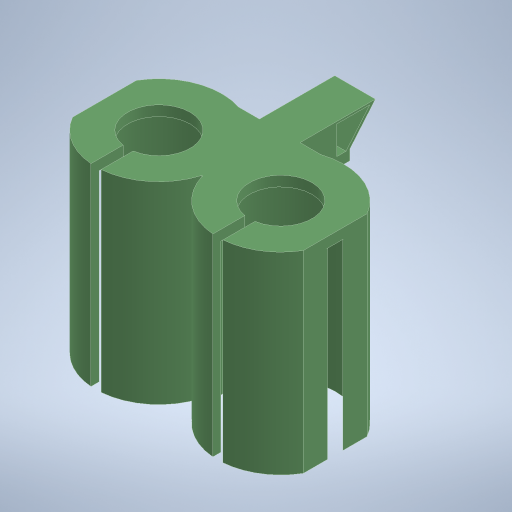
# Autodesk Inventor part: vialHolder_2v
Saved by Autodesk Inventor 2023.4 (Build 274418000, 418)
## iProperties
Created: 2023-09-01
Part Number: vialHolder_2v
Material: Generic
Document SubType Name: Modeling
Designer: SB13FLLT004
Density: 1 g/cm^3
Appearance: Dark Green(3)
Author: SB13FLLT004
Autodesk Inventor part; units mm, degrees
ref_plane "YZ Plane" through (0, 0, 0) normal (1, 0, 0) x (0, 1, 0)
ref_plane "XZ Plane" through (0, 0, 0) normal (0, 1, 0) x (-1, 0, 0)
ref_plane "XY Plane" through (0, 0, 0) normal (0, 0, 1) x (1, 0, 0)
derived "main_manifold_8v_v02.ipt"
sketch "Sketch:MM: flow sensor" plane through (0, 0, -27.94) normal (0, -1, 0) x (1, 0, 0)
  line L0 (19.2278, 23.241) -> (22.6822, 23.241)
  line L1 (49.7078, 23.241) -> (53.1622, 23.241)
  line L2 (110.6678, 23.241) -> (114.1222, 23.241)
  line L3 (80.1878, 23.241) -> (83.6422, 23.241)
  line L4 (141.1478, 23.241) -> (144.6022, 23.241)
  line L5 (171.6278, 23.241) -> (175.0822, 23.241)
  line L6 (202.1078, 23.241) -> (205.5622, 23.241)
  line L7 (232.5878, 23.241) -> (236.0422, 23.241)
  line L8 (0, 27.94) -> (247.65, 27.94)
  point P0 (20.955, 23.241)
  point P1 (51.435, 23.241)
  point P2 (51.435, 23.241)
  point P3 (20.955, 23.241)
  point P4 (81.915, 23.241)
  point P5 (112.395, 23.241)
  point P6 (81.915, 23.241)
  point P7 (112.395, 23.241)
  point P8 (142.875, 23.241)
  point P9 (173.355, 23.241)
  point P10 (203.835, 23.241)
  point P11 (234.315, 23.241)
  point P12 (142.875, 23.241)
  point P13 (173.355, 23.241)
  point P14 (203.835, 23.241)
  point P15 (234.315, 23.241)
derived "vial_ST_01.ipt"
derived "mainPlate.ipt"
sketch "Sketch:VH: vials" plane through (0, 0, 0) normal (0, 1, 0) x (-1, 0, 0)
  circle A0 centre (-20.955, -4.699) radius 15.7798
  circle A1 centre (-20.955, -4.699) radius 13.7477
  circle A2 centre (-20.955, -4.699) radius 7.5565 construction
  circle A3 centre (-20.955, -4.699) radius 7.8105
  circle A4 centre (-51.435, -4.699) radius 15.7798
  circle A5 centre (-51.435, -4.699) radius 13.7477
  circle A6 centre (-51.435, -4.699) radius 7.8105
  line L0 (-36.0958, -9.144) -> (-36.2942, -9.144)
  line L1 (-36.0958, -0.254) -> (-36.2942, -0.254)
  point P0 (0, 0)
  point P1 (-36.195, -0.6072)
  point P2 (-36.195, -8.7908)
  dimension "cap_diameter" = 15.113
  dimension "d5" = 15.621
  dimension "extra_space_around_vial_front_and_back" = 4.445
  constraints: 7 centre point, 7 coincident, 4 end point, 4 point on circle, 3 equal radius, 2 vertical alignment, 1 concentric, 1 horizontal, 1 horizontal alignment, 1 other
  measures "cap_diameter" diameter of A2
  measures "d5" diameter of A3
  measures "extra_space_around_vial_front_and_back" vertical distance of A0.centre L1.start
sketch "Sketch:VH: side cutout" plane through (0, 0, 0) normal (0, 1, 0) x (-1, 0, 0)
  line L0 (-7.3399, -12.6758) -> (-7.3399, 3.2778)
  line L1 (-65.0501, -12.6758) -> (-65.0501, 3.2778)
  circle A0 centre (-51.435, -4.699) radius 15.7798 projected
  circle A1 centre (-51.435, -4.699) radius 13.7477 projected
  circle A2 centre (-20.955, -4.699) radius 15.7798 projected
  circle A3 centre (-20.955, -4.699) radius 13.7477 projected
  line L2 (-5.4104, -7.4129) -> (-7.4778, -7.4129) construction
  line L3 (-5.4104, -1.9851) -> (-7.4778, -1.9851) construction
  line L4 (-7.4778, -7.4129) -> (-7.4778, -1.9851) construction
  point P0 (0, 0)
  point P1 (-7.3399, -6.604)
  point P2 (-7.3399, -2.794)
  point P3 (-7.4778, -4.699)
  dimension "d12" = 13.6151
  dimension "d57" = 3.81
  dimension "d58" = 5.4278
  constraints: 10 end point, 10 point on circle, 3 horizontal alignment, 2 point on line, 1 midpoint, 1 parallel, 1 perpendicular, 1 vertical
  measures "d12" distance from line of A2.centre L0
  measures "d57" distance of A3.end A3.start
  measures "d58" distance of L2.end L3.end
extrude "Ex: top of vials" add sketch "Sketch:VH: vials" along normal blind 2.54 contours A0 A4 | A0 A4 L1 | L0 A4 A0 | A4 A0 | A0 A4 | A1 | A5
extrude "Ex: around vials" add sketch "Sketch:VH: vials" against normal blind 45.72 contours A0 A4 | A0 A4 L1 | L0 A4 A0 | A4 A0 | A0 A4
extrude "Ex: side cutout" cut sketch "Sketch:VH: side cutout" along normal through all both and the other way through all contours L0 A3 A2 | L0 A3 | A0 L1 A1 | A1 L1 picked at (-7.3154, -5.1231) picked at (-65.0894, -4.4867)
sketch "Sketch:VH: screw part" plane through (0, 2.54, 0) normal (0, 1, 0) x (-1, 0, 0)
  circle A0 centre (-20.955, -4.699) radius 15.7798 projected
  circle A1 centre (-51.435, -4.699) radius 15.7798 projected
  line L0 (-16.0074, -19.6831) -> (-56.3826, -19.6831)
  line L1 (-36.0958, -9.144) -> (-36.2942, -9.144) projected
  line L2 (-31.115, -19.6831) -> (-31.115, -28.916)
  line L3 (-31.115, -28.916) -> (-41.275, -28.916)
  line L4 (-41.275, -28.916) -> (-41.275, -19.6831)
  line L5 (-33.9979, -28.916) -> (-38.3921, -28.916) construction
  line L6 (-38.3921, -28.916) -> (-38.3921, -23.582) construction
  line L7 (-38.3921, -23.582) -> (-33.9979, -23.582) construction
  line L8 (-33.9979, -23.582) -> (-33.9979, -28.916) construction
  point P0 (0, 0)
  point P1 (-36.195, -19.6831)
  point P2 (-36.195, -9.144)
  point P3 (-36.195, -28.916)
  point P4 (-25.9026, -19.6831)
  point P5 (-46.4874, -19.6831)
  dimension "d15" = 10.16
  dimension "d18" = 9.2329
  constraints: 16 end point, 6 perpendicular, 4 midpoint, 3 vertical alignment, 2 horizontal, 2 point on circle, 2 point on line, 1 collinear, 1 horizontal alignment
  measures "d15" distance of L2.end L3.end
  measures "d18" distance of L3.end L4.end
extrude "Ex: screw area" add sketch "Sketch:VH: screw part" against normal blind 7.62 contours L0 A1 L1 A0 | L2 L3 L4 L0
sketch "Sketch:VH: screw hole" plane through (41.275, 2.54, -28.916) normal (0, 0, -1) x (-1, 0, 0)
  line L0 (0, 0) -> (10.16, 0) projected
  line L1 (10.16, -7.62) -> (0, -7.62) projected
  line L2 (0, -7.62) -> (0, -7.62)
  line L3 (0, -7.62) -> (10.16, -7.62)
  line L4 (10.16, -7.62) -> (10.16, -7.62)
  point P0 (41.275, -2.54)
  point P1 (5.08, -3.175)
  point P2 (5.08, 0)
  dimension "d72" = 3.175
  dimension "screwhole_to_btm_of_MP" = 4.445
  constraints: 6 end point, 2 perpendicular, 1 collinear, 1 midpoint, 1 vertical alignment
  measures "d72" distance from line of L0 point (5.08, -3.175)
  measures "screwhole_to_btm_of_MP" distance from line of L3 point (5.08, -3.175)
hole "Hole: screw to MP" at (36.195, -0.635, -28.916) direction (0, 0, 1) diameter 4.3942 depth 5.334
sketch "Sketch:VH: extend front" plane through (0, 0, 0) normal (0, 1, 0) x (-1, 0, 0)
  arc A0 (-7.3399, 4.2408) -> (-36.6245, -0.254) centre (-20.955, -4.699) ccw
  circle A1 centre (-20.955, -4.699) radius 15.7798 projected
  line L0 (-7.3399, -12.6758) -> (-7.3399, 3.2778) projected
  line L1 (-36.0958, -0.254) -> (-36.2942, -0.254) projected
  line L2 (-7.3399, 3.2778) -> (-7.3399, 4.2408)
  circle A2 centre (-51.435, -4.699) radius 15.7798 projected
  line L3 (-65.0501, -12.6758) -> (-65.0501, 3.2778) projected
  arc A3 (-35.7655, -0.254) -> (-65.0501, 4.2408) centre (-51.435, -4.699) ccw
  line L4 (-65.0501, 4.2408) -> (-65.0501, 3.2778)
  point P0 (0, 0)
  dimension "d47" = 0.508
  constraints: 4 end point, 4 point on circle, 2 centre point, 2 collinear, 2 concentric, 2 point on line, 1 equal radius
  measures "d47" radial gap between concentric circles of A0 A1
sketch "Sketch:VH: front cutout" plane through (0, 0, 0) normal (0, 1, 0) x (-1, 0, 0)
  line L0 (-19.685, -19.886) -> (-19.685, 11.5392)
  line L1 (-22.225, -19.886) -> (-22.225, 11.5392)
  circle A0 centre (-20.955, -4.699) radius 13.7477 projected
  circle A1 centre (-51.435, -4.699) radius 13.7477 projected
  circle A2 centre (-20.955, -4.699) radius 7.8105 projected
  circle A3 centre (-51.435, -4.699) radius 7.8105 projected
  line L2 (-19.685, -4.699) -> (-22.225, -4.699) construction
  line L3 (-50.165, -19.6311) -> (-50.165, 11.5392)
  line L4 (-52.705, -19.6311) -> (-52.705, 11.5392)
  line L5 (-50.165, -4.699) -> (-52.705, -4.699) construction
  line L6 (-36.0958, -0.254) -> (-36.2942, -0.254) projected
  arc A4 (-7.3399, 4.2408) -> (-36.6245, -0.254) centre (-20.955, -4.699) ccw projected
  arc A5 (-35.7655, -0.254) -> (-65.0501, 4.2408) centre (-51.435, -4.699) ccw projected
  point P0 (0, 0)
  point P1 (-22.225, 3.0076)
  point P2 (-19.685, 3.0076)
  point P3 (-19.685, 8.99)
  point P4 (-22.225, 8.99)
  point P5 (-52.705, 3.0076)
  point P6 (-50.165, 3.0076)
  point P7 (-22.225, -18.388)
  point P8 (-19.685, -18.388)
  point P9 (-52.705, -12.4056)
  point P10 (-50.165, -12.4056)
  dimension "d44" = 2.54
  constraints: 12 end point, 4 point on circle, 4 point on line, 3 parallel, 2 coincident, 2 collinear, 2 midpoint, 1 horizontal, 1 vertical
  measures "d44" distance between parallel lines of L1 L0
extrude "Ex: front cutout" cut sketch "Sketch:VH: front cutout" along normal through all both and the other way through all contours A2 L1 A0 L0 | L1 A4 L0 A0 | L3 A3 L4 A1 | A1 L4 A5 L3 picked at (-19.9667, 5.0325) picked at (-50.4467, 5.0325)
sketch "Sketch: under MP" plane through (0, -5.08, 0) normal (0, 1, 0) x (-1, 0, 0)
  line L0 (-31.115, -19.6831) -> (-31.115, -28.916) projected
  line L1 (-31.115, -28.916) -> (-41.275, -28.916) projected
  line L2 (-41.275, -28.916) -> (-41.275, -19.6831) projected
  line L3 (-16.0074, -19.6831) -> (-56.3826, -19.6831) projected
  circle A0 centre (-20.955, -4.699) radius 15.7798 projected
  circle A1 centre (-51.435, -4.699) radius 15.7798 projected
  line L4 (-31.115, -28.916) -> (-31.115, -32.1164)
  line L5 (-31.115, -32.1164) -> (-41.275, -32.1164)
  line L6 (-41.275, -32.1164) -> (-41.275, -28.916)
  point P0 (0, 0)
  point P1 (-36.195, -8.7908)
  point P2 (-46.4874, -19.6831)
  point P3 (-25.9026, -19.6831)
  dimension "d77" = 3.2004
  constraints: 6 end point, 2 perpendicular, 1 parallel, 2 other
  measures "d77" distance of L5.end L1.end
extrude "Ex: under MP" add sketch "Sketch: under MP" against normal blind 2.54 contours L0 L1 L2 L3 | L3 A1 A0 | L4 L5 L6 L1 picked at (-37.4519, -18.301)
sketch "Sketch12" plane through (31.115, 2.54, -28.916) normal (-1, 0, 0) x (0, 0, 1)
  line L0 (0, -0.54) -> (-8.2013, -0.54)
  line L1 (-8.2013, -0.54) -> (-2.2605, -7.62)
  line L2 (0, 0) -> (-9.5943, 0)
  line L3 (-9.5943, 0) -> (-3.2004, -7.62)
  line L4 (0, 0) -> (0, -7.62) projected
  line L5 (-3.2004, -7.62) -> (-3.2004, -7.62) construction
  line L6 (-3.2004, -7.62) -> (0, -7.62) projected
  line L7 (-1.0693, -7.62) -> (-1.0693, 0) construction
  line L8 (0, -5.3721) -> (0, -0.9779) construction
  line L9 (0, -0.9779) -> (-8.7738, -0.9779) construction
  point P0 (28.916, -2.54)
  point P1 (-1.6002, -7.62)
  dimension "d78" = 50
  dimension "d79" = 1.0693
  dimension "d82" = 0.9399
  dimension "d85" = 0.54
  dimension "d86" = 0.72
  dimension "d87" = 0.4379
  dimension "d89" = 6.6011
  dimension "d90" = 7.08
  dimension "d91" = 2.2605
  constraints: 14 end point, 6 point on line, 2 coincident, 2 horizontal, 2 parallel, 1 collinear, 1 midpoint, 1 vertical
  measures "d78" angle of L0 L1
  measures "d79" distance between parallel lines of L7 L4
  measures "d82" distance of L3.end L1.end
  measures "d85" distance between parallel lines of L2 L0
  measures "d86" distance between parallel lines of L3 L1
  measures "d87" distance between parallel lines of L0 L9
  measures "d89" horizontal distance of L0.end point (-1.6, -7.62)
  measures "d90" vertical distance of L1.end L0.end
  measures "d91" distance from line of L4 L1.end
extrude "Extrusion12" add sketch "Sketch12" against normal up to surface (10.16 mm away) contours L0 L1 L6 L3 L2 L4
equation "\"cap_diameter\" = 2 * cap_radius_inner"
equation "\"cap_radius_inner\" = 7.5565"
body "Solid1"
